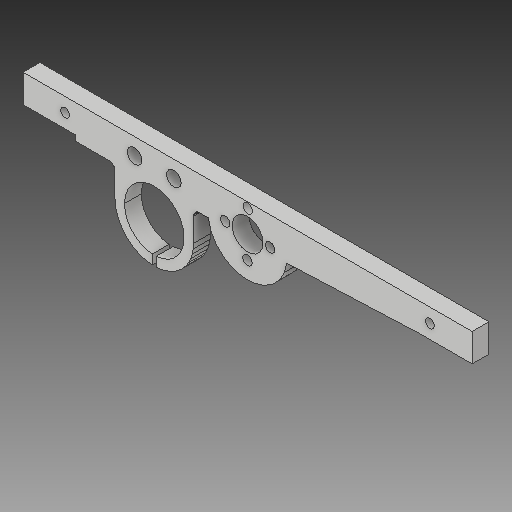
# Autodesk Inventor part: Rear-Bed-Holder-mid
Saved by Autodesk Inventor 2017 (Build 210142000, 142)
## iProperties
Created: 2016-07-12
Part Number: Rear-Bed-Holder-mid
Material: Generic
Document SubType Name: Modeling
Designer: joshmamo
Density: 1 g/cm^3
Appearance: Default
Author: joshmamo
Autodesk Inventor part; units mm, degrees
ref_plane "YZ Plane" through (0, 0, 0) normal (1, 0, 0) x (0, 1, 0)
ref_plane "XZ Plane" through (0, 0, 0) normal (0, 1, 0) x (-1, 0, 0)
ref_plane "XY Plane" through (0, 0, 0) normal (0, 0, 1) x (1, 0, 0)
sketch "Sketch1" plane through (0, 0, 0) normal (0, 0, 1) x (1, 0, 0)
  line L0 (326.8705, 297.7695) -> (327.1965, 298.0306)
  line L1 (327.1965, 298.0306) -> (327.4439, 298.3671)
  line L2 (327.4439, 298.3671) -> (327.5957, 298.7562)
  line L3 (327.5957, 298.7562) -> (327.6417, 299.1714)
  line L4 (327.6417, 299.1714) -> (327.5786, 299.5843)
  line L5 (324.4883, 299.5205) -> (324.4424, 299.1053)
  line L6 (324.4424, 299.1053) -> (324.5054, 298.6924)
  line L7 (324.5054, 298.6924) -> (324.6732, 298.3099)
  line L8 (324.6732, 298.3099) -> (324.9342, 297.9839)
  line L9 (324.9342, 297.9839) -> (325.2708, 297.7365)
  line L10 (325.2708, 297.7365) -> (325.6599, 297.5847)
  line L11 (325.6599, 297.5847) -> (326.075, 297.5387)
  line L12 (326.075, 297.5387) -> (326.4879, 297.6017)
  line L13 (326.4879, 297.6017) -> (326.8705, 297.7695)
  line L14 (327.2625, 278.7736) -> (327.5885, 279.0346)
  line L15 (327.5885, 279.0346) -> (327.8359, 279.3712)
  line L16 (327.8359, 279.3712) -> (327.9877, 279.7603)
  line L17 (327.9877, 279.7603) -> (328.0337, 280.1754)
  line L18 (328.0337, 280.1754) -> (327.9707, 280.5883)
  line L19 (327.9707, 280.5883) -> (327.8029, 280.9708)
  line L20 (327.8029, 280.9708) -> (327.5418, 281.2969)
  line L21 (327.5418, 281.2969) -> (327.2053, 281.5442)
  line L22 (327.2053, 281.5442) -> (326.8162, 281.6961)
  line L23 (326.8162, 281.6961) -> (326.401, 281.7421)
  line L24 (326.401, 281.7421) -> (325.9881, 281.679)
  line L25 (325.9881, 281.679) -> (325.6056, 281.5112)
  line L26 (325.6056, 281.5112) -> (325.2796, 281.2502)
  line L27 (325.2796, 281.2502) -> (325.0322, 280.9136)
  line L28 (325.0322, 280.9136) -> (324.8804, 280.5245)
  line L29 (324.8804, 280.5245) -> (324.8344, 280.1094)
  line L30 (324.8344, 280.1094) -> (324.8974, 279.6965)
  line L31 (324.8974, 279.6965) -> (325.0652, 279.314)
  line L32 (325.0652, 279.314) -> (325.3263, 278.9879)
  line L33 (325.3263, 278.9879) -> (325.6628, 278.7405)
  line L34 (325.6628, 278.7405) -> (326.0519, 278.5887)
  line L35 (326.0519, 278.5887) -> (326.4671, 278.5427)
  line L36 (326.4671, 278.5427) -> (326.88, 278.6058)
  line L37 (326.88, 278.6058) -> (327.2625, 278.7736)
  line L38 (262.6237, 293.8404) -> (262.7835, 294.2263)
  line L39 (262.7835, 294.2263) -> (262.838, 294.6404)
  line L40 (262.838, 294.6404) -> (262.7835, 295.0545)
  line L41 (262.7835, 295.0545) -> (262.6237, 295.4404)
  line L42 (262.6237, 295.4404) -> (262.3694, 295.7717)
  line L43 (262.3694, 295.7717) -> (262.038, 296.026)
  line L44 (262.038, 296.026) -> (261.6522, 296.1859)
  line L45 (261.6522, 296.1859) -> (261.238, 296.2404)
  line L46 (261.238, 296.2404) -> (260.8239, 296.1859)
  line L47 (260.8239, 296.1859) -> (260.438, 296.026)
  line L48 (260.438, 296.026) -> (260.1067, 295.7717)
  line L49 (260.1067, 295.7717) -> (259.8524, 295.4404)
  line L50 (259.8524, 295.4404) -> (259.6926, 295.0545)
  line L51 (259.6926, 295.0545) -> (259.638, 294.6404)
  line L52 (259.638, 294.6404) -> (259.6926, 294.2263)
  line L53 (259.6926, 294.2263) -> (259.8524, 293.8404)
  line L54 (259.8524, 293.8404) -> (260.1067, 293.509)
  line L55 (260.1067, 293.509) -> (260.438, 293.2547)
  line L56 (260.438, 293.2547) -> (260.8239, 293.0949)
  line L57 (260.8239, 293.0949) -> (261.238, 293.0404)
  line L58 (261.238, 293.0404) -> (261.6522, 293.0949)
  line L59 (261.6522, 293.0949) -> (262.038, 293.2547)
  line L60 (262.038, 293.2547) -> (262.3694, 293.509)
  line L61 (262.3694, 293.509) -> (262.6237, 293.8404)
  line L62 (390.8239, 296.1859) -> (390.438, 296.026)
  line L63 (390.438, 296.026) -> (390.1067, 295.7717)
  line L64 (390.1067, 295.7717) -> (389.8524, 295.4404)
  line L65 (389.8524, 295.4404) -> (389.6926, 295.0545)
  line L66 (389.6926, 295.0545) -> (389.638, 294.6404)
  line L67 (389.638, 294.6404) -> (389.6926, 294.2263)
  line L68 (389.6926, 294.2263) -> (389.8524, 293.8404)
  line L69 (389.8524, 293.8404) -> (390.1067, 293.509)
  line L70 (390.1067, 293.509) -> (390.438, 293.2547)
  line L71 (390.438, 293.2547) -> (390.8239, 293.0949)
  line L72 (390.8239, 293.0949) -> (391.238, 293.0404)
  line L73 (391.238, 293.0404) -> (391.6522, 293.0949)
  line L74 (391.6522, 293.0949) -> (392.038, 293.2547)
  line L75 (392.038, 293.2547) -> (392.3694, 293.509)
  line L76 (392.3694, 293.509) -> (392.6237, 293.8404)
  line L77 (392.6237, 293.8404) -> (392.7835, 294.2263)
  line L78 (392.7835, 294.2263) -> (392.838, 294.6404)
  line L79 (392.838, 294.6404) -> (392.7835, 295.0545)
  line L80 (392.7835, 295.0545) -> (392.6237, 295.4404)
  line L81 (392.6237, 295.4404) -> (392.3694, 295.7717)
  line L82 (392.3694, 295.7717) -> (392.038, 296.026)
  line L83 (392.038, 296.026) -> (391.6522, 296.1859)
  line L84 (391.6522, 296.1859) -> (391.238, 296.2404)
  line L85 (391.238, 296.2404) -> (390.8239, 296.1859)
  line L86 (318.1419, 288.6731) -> (318.2938, 289.0622)
  line L87 (318.2938, 289.0622) -> (318.3397, 289.4774)
  line L88 (318.3397, 289.4774) -> (318.2767, 289.8903)
  line L89 (318.2767, 289.8903) -> (318.1089, 290.2728)
  line L90 (318.1089, 290.2728) -> (317.8479, 290.5988)
  line L91 (317.8479, 290.5988) -> (317.5113, 290.8462)
  line L92 (317.5113, 290.8462) -> (317.1222, 290.9981)
  line L93 (317.1222, 290.9981) -> (316.7071, 291.044)
  line L94 (316.7071, 291.044) -> (316.2942, 290.981)
  line L95 (316.2942, 290.981) -> (315.9116, 290.8132)
  line L96 (315.9116, 290.8132) -> (315.5856, 290.5521)
  line L97 (315.5856, 290.5521) -> (315.3382, 290.2156)
  line L98 (315.3382, 290.2156) -> (315.1864, 289.8265)
  line L99 (315.1864, 289.8265) -> (315.1404, 289.4114)
  line L100 (315.1404, 289.4114) -> (315.2035, 288.9985)
  line L101 (315.2035, 288.9985) -> (315.3712, 288.6159)
  line L102 (315.3712, 288.6159) -> (315.6323, 288.2899)
  line L103 (315.6323, 288.2899) -> (315.9688, 288.0425)
  line L104 (315.9688, 288.0425) -> (316.3579, 287.8907)
  line L105 (316.3579, 287.8907) -> (316.7731, 287.8447)
  line L106 (316.7731, 287.8447) -> (317.186, 287.9078)
  line L107 (317.186, 287.9078) -> (317.5685, 288.0755)
  line L108 (317.5685, 288.0755) -> (317.8945, 288.3366)
  line L109 (317.8945, 288.3366) -> (318.1419, 288.6731)
  line L110 (334.1994, 289.3905) -> (334.3672, 289.008)
  line L111 (334.3672, 289.008) -> (334.6282, 288.6819)
  line L112 (334.6282, 288.6819) -> (334.9648, 288.4345)
  line L113 (334.9648, 288.4345) -> (335.3539, 288.2827)
  line L114 (335.3539, 288.2827) -> (335.769, 288.2367)
  line L115 (335.769, 288.2367) -> (336.1819, 288.2998)
  line L116 (336.1819, 288.2998) -> (336.5644, 288.4675)
  line L117 (336.5644, 288.4675) -> (336.8905, 288.7286)
  line L118 (336.8905, 288.7286) -> (337.1379, 289.0651)
  line L119 (337.1379, 289.0651) -> (337.2897, 289.4542)
  line L120 (337.2897, 289.4542) -> (337.3357, 289.8694)
  line L121 (337.3357, 289.8694) -> (337.2726, 290.2823)
  line L122 (337.2726, 290.2823) -> (337.1049, 290.6648)
  line L123 (337.1049, 290.6648) -> (336.8438, 290.9908)
  line L124 (336.8438, 290.9908) -> (336.5073, 291.2382)
  line L125 (336.5073, 291.2382) -> (336.1182, 291.3901)
  line L126 (336.1182, 291.3901) -> (335.703, 291.436)
  line L127 (335.703, 291.436) -> (335.2901, 291.373)
  line L128 (335.2901, 291.373) -> (334.9076, 291.2052)
  line L129 (334.9076, 291.2052) -> (334.5815, 290.9442)
  line L130 (334.5815, 290.9442) -> (334.3342, 290.6076)
  line L131 (334.3342, 290.6076) -> (334.1823, 290.2185)
  line L132 (334.1823, 290.2185) -> (334.1364, 289.8034)
  line L133 (334.1364, 289.8034) -> (334.1994, 289.3905)
  line L134 (324.6214, 275.5909) -> (321.0402, 276.4881)
  line L135 (321.0402, 276.4881) -> (317.8133, 278.2815)
  line L136 (317.8133, 278.2815) -> (315.1604, 280.8491)
  line L137 (315.1604, 280.8491) -> (313.2626, 284.0157)
  line L138 (313.2626, 284.0157) -> (312.2489, 287.5657)
  line L139 (312.2489, 287.5657) -> (312.2467, 287.7002)
  line L140 (312.2467, 287.7002) -> (309.0912, 287.7002)
  line L141 (309.0912, 287.7002) -> (308.7265, 287.6683)
  line L142 (308.7265, 287.6683) -> (308.373, 287.5736)
  line L143 (308.373, 287.5736) -> (308.0412, 287.4189)
  line L144 (308.0412, 287.4189) -> (307.7413, 287.2089)
  line L145 (307.7413, 287.2089) -> (307.4825, 286.9501)
  line L146 (307.4825, 286.9501) -> (307.2725, 286.6502)
  line L147 (307.2725, 286.6502) -> (307.1178, 286.3185)
  line L148 (307.1178, 286.3185) -> (307.0231, 285.9649)
  line L149 (307.0231, 285.9649) -> (306.9912, 285.6002)
  line L150 (306.9912, 285.6002) -> (306.9912, 277.2002)
  line L151 (306.9912, 277.2002) -> (306.8789, 275.4307)
  line L152 (306.8789, 275.4307) -> (306.5439, 273.6896)
  line L153 (306.5439, 273.6896) -> (305.9915, 272.0048)
  line L154 (305.9915, 272.0048) -> (305.2306, 270.4034)
  line L155 (305.2306, 270.4034) -> (304.2733, 268.9109)
  line L156 (304.2733, 268.9109) -> (303.1352, 267.5514)
  line L157 (303.1352, 267.5514) -> (301.8343, 266.3467)
  line L158 (301.8343, 266.3467) -> (300.3915, 265.316)
  line L159 (300.3915, 265.316) -> (298.8301, 264.476)
  line L160 (298.8301, 264.476) -> (297.175, 263.84)
  line L161 (297.175, 263.84) -> (295.4529, 263.4184)
  line L162 (295.4529, 263.4184) -> (293.6912, 263.2177)
  line L163 (293.6912, 263.2177) -> (293.6912, 266.7236)
  line L164 (293.6912, 266.7236) -> (295.3277, 266.9635)
  line L165 (295.3277, 266.9635) -> (296.9062, 267.4574)
  line L166 (296.9062, 267.4574) -> (298.3876, 268.1931)
  line L167 (298.3876, 268.1931) -> (299.7351, 269.1522)
  line L168 (299.7351, 269.1522) -> (300.9152, 270.3111)
  line L169 (300.9152, 270.3111) -> (301.8987, 271.6409)
  line L170 (301.8987, 271.6409) -> (302.6612, 273.1086)
  line L171 (302.6612, 273.1086) -> (303.1837, 274.6779)
  line L172 (303.1837, 274.6779) -> (303.4534, 276.3098)
  line L173 (303.4534, 276.3098) -> (303.4634, 277.9637)
  line L174 (303.4634, 277.9637) -> (303.2136, 279.5988)
  line L175 (303.2136, 279.5988) -> (302.7101, 281.1743)
  line L176 (302.7101, 281.1743) -> (301.9655, 282.6511)
  line L177 (301.9655, 282.6511) -> (300.9982, 283.9928)
  line L178 (300.9982, 283.9928) -> (299.8322, 285.1659)
  line L179 (299.8322, 285.1659) -> (298.4964, 286.1413)
  line L180 (298.4964, 286.1413) -> (297.0241, 286.8949)
  line L181 (297.0241, 286.8949) -> (295.4517, 287.4079)
  line L182 (295.4517, 287.4079) -> (293.8182, 287.6676)
  line L183 (293.8182, 287.6676) -> (292.1642, 287.6676)
  line L184 (292.1642, 287.6676) -> (290.5307, 287.4079)
  line L185 (290.5307, 287.4079) -> (288.9583, 286.8949)
  line L186 (288.9583, 286.8949) -> (287.486, 286.1413)
  line L187 (287.486, 286.1413) -> (286.1502, 285.1659)
  line L188 (286.1502, 285.1659) -> (284.9842, 283.9928)
  line L189 (284.9842, 283.9928) -> (284.0169, 282.6511)
  line L190 (284.0169, 282.6511) -> (283.2723, 281.1743)
  line L191 (283.2723, 281.1743) -> (282.7688, 279.5988)
  line L192 (282.7688, 279.5988) -> (282.519, 277.9637)
  line L193 (282.519, 277.9637) -> (282.529, 276.3098)
  line L194 (282.529, 276.3098) -> (282.7986, 274.6779)
  line L195 (282.7986, 274.6779) -> (283.3212, 273.1086)
  line L196 (283.3212, 273.1086) -> (284.0837, 271.6409)
  line L197 (284.0837, 271.6409) -> (285.0672, 270.3111)
  line L198 (285.0672, 270.3111) -> (286.2473, 269.1522)
  line L199 (286.2473, 269.1522) -> (287.5948, 268.1931)
  line L200 (287.5948, 268.1931) -> (289.0762, 267.4574)
  line L201 (289.0762, 267.4574) -> (290.6547, 266.9635)
  line L202 (290.6547, 266.9635) -> (292.2912, 266.7236)
  line L203 (292.2912, 266.7236) -> (292.2912, 263.2177)
  line L204 (292.2912, 263.2177) -> (290.5295, 263.4184)
  line L205 (290.5295, 263.4184) -> (288.8073, 263.84)
  line L206 (288.8073, 263.84) -> (287.1523, 264.476)
  line L207 (287.1523, 264.476) -> (285.5909, 265.316)
  line L208 (285.5909, 265.316) -> (284.1481, 266.3467)
  line L209 (284.1481, 266.3467) -> (282.8472, 267.5514)
  line L210 (282.8472, 267.5514) -> (281.709, 268.9109)
  line L211 (281.709, 268.9109) -> (280.7518, 270.4034)
  line L212 (280.7518, 270.4034) -> (279.9909, 272.0048)
  line L213 (279.9909, 272.0048) -> (279.4385, 273.6896)
  line L214 (279.4385, 273.6896) -> (279.1035, 275.4307)
  line L215 (279.1035, 275.4307) -> (278.9912, 277.2002)
  line L216 (278.9912, 277.2002) -> (278.9912, 285.6002)
  line L217 (278.9912, 285.6002) -> (278.9593, 285.9649)
  line L218 (278.9593, 285.9649) -> (278.8645, 286.3185)
  line L219 (278.8645, 286.3185) -> (278.7098, 286.6502)
  line L220 (278.7098, 286.6502) -> (278.4999, 286.9501)
  line L221 (278.4999, 286.9501) -> (278.241, 287.2089)
  line L222 (278.241, 287.2089) -> (277.9412, 287.4189)
  line L223 (277.9412, 287.4189) -> (277.6094, 287.5736)
  line L224 (277.6094, 287.5736) -> (277.2559, 287.6683)
  line L225 (277.2559, 287.6683) -> (276.8912, 287.7002)
  line L226 (276.8912, 287.7002) -> (264.9912, 287.7002)
  line L227 (264.9912, 287.7002) -> (264.9912, 289.6404)
  line L228 (264.9912, 289.6404) -> (246.238, 289.6404)
  line L229 (246.238, 289.6404) -> (246.238, 299.6404)
  line L230 (246.238, 299.6404) -> (406.238, 299.6404)
  line L231 (406.238, 299.6404) -> (406.238, 289.6404)
  line L232 (406.238, 289.6404) -> (387.4849, 289.6404)
  line L233 (387.4849, 289.6404) -> (340.2064, 287.7002)
  line L234 (340.2064, 287.7002) -> (339.3903, 284.4425)
  line L235 (339.3903, 284.4425) -> (337.5969, 281.2156)
  line L236 (337.5969, 281.2156) -> (335.0293, 278.5628)
  line L237 (335.0293, 278.5628) -> (331.8627, 276.6649)
  line L238 (331.8627, 276.6649) -> (328.3127, 275.6512)
  line L239 (328.3127, 275.6512) -> (324.6214, 275.5909)
  circle A0 centre (326.238, 289.6404) radius 5.5
  circle A1 centre (285.9912, 293.6676) radius 2.6
  circle A2 centre (299.9912, 293.6676) radius 2.6
  point P0 (0, 0)
  constraints: 480 end point, 3 centre point
extrude "Extrusion1" add sketch "Sketch1" along normal blind 6
sketch "Sketch2" plane through (0, 0, 6) normal (0, 0, 1) x (1, 0, 0)
  line L0 (318.3397, 289.4774) -> (318.2938, 289.0622) projected
  line L1 (315.1404, 289.4114) -> (318.3397, 289.4774)
  line L2 (334.1823, 290.2185) -> (334.1364, 289.8034) projected
  line L3 (337.2726, 290.2823) -> (337.3357, 289.8694) projected
  line L4 (334.1364, 289.8034) -> (337.3357, 289.8694)
  line L5 (318.2767, 289.8903) -> (318.3397, 289.4774) projected
  line L6 (334.1364, 289.8034) -> (318.3397, 289.4774)
  line L7 (324.8804, 280.5245) -> (324.8344, 280.1094) projected
  line L8 (328.0337, 280.1754) -> (324.8344, 280.1094)
  circle A0 centre (326.434, 280.1424) radius 1.6
  circle A1 centre (326.042, 299.1383) radius 1.6
  point P0 (0, 0)
  dimension "d2" = 3.2
  constraints: 8 end point, 2 centre point, 1 midpoint, 1 symmetric about line, 1 other
  measures "d2" diameter of A0
extrude "Extrusion2" cut sketch "Sketch2" against normal through all contours A1
sketch "Sketch3" plane through (0, 0, 6) normal (0, 0, 1) x (1, 0, 0)
  line L0 (262.7835, 295.0545) -> (262.838, 294.6404) projected
  line L1 (259.6926, 294.2263) -> (259.638, 294.6404) projected
  line L2 (262.838, 294.6404) -> (259.638, 294.6404)
  line L3 (389.638, 294.6404) -> (389.6926, 294.2263) projected
  line L4 (392.838, 294.6404) -> (389.638, 294.6404)
  point P0 (0, 0)
  point P1 (391.238, 294.6404)
  point P2 (261.238, 294.6404)
  constraints: 4 end point, 2 horizontal, 2 midpoint
hole "Hole1" at (391.238, 294.6404, 6) at (261.238, 294.6404, 6) direction (0, 0, -1) diameter 3.2 depth 8 tip angle 118
sketch "Sketch4" plane through (0, 0, 6) normal (0, 0, 1) x (1, 0, 0)
  line L0 (303.4634, 277.9637) -> (303.4534, 276.3098) projected
  line L1 (303.4584, 277.1368) -> (282.524, 277.1368)
  line L2 (282.519, 277.9637) -> (282.529, 276.3098) projected
  point P0 (0, 0)
  point P1 (292.9912, 277.1368)
  constraints: 3 midpoint, 2 end point
hole "Hole2" at (292.9912, 277.1368, 6) direction (0, 0, -1) diameter 21.2 depth 8 tip angle 118
sketch "Sketch5" plane through (0, 0, 6) normal (0, 0, 1) x (1, 0, 0)
  arc A0 (293.6912, 266.6865) -> (292.2912, 266.6865) centre (292.9912, 277.2634) ccw projected
  point P0 (0, 0)
hole "Hole3" at (292.9912, 277.2634, 6) direction (0, 0, -1) diameter 21.2 depth 8 tip angle 118
sketch "Sketch6" plane through (0, 0, 6) normal (0, 0, 1) x (1, 0, 0)
  line L0 (337.2726, 290.2823) -> (337.3357, 289.8694) projected
  line L1 (334.1994, 289.3905) -> (334.1364, 289.8034) projected
  line L2 (337.3357, 289.8694) -> (334.1364, 289.8034)
  line L3 (327.9707, 280.5883) -> (328.0337, 280.1754) projected
  line L4 (324.8344, 280.1094) -> (324.8804, 280.5245) projected
  line L5 (328.0337, 280.1754) -> (324.8344, 280.1094)
  line L6 (318.3397, 289.4774) -> (318.2938, 289.0622) projected
  line L7 (315.2035, 288.9985) -> (315.1404, 289.4114) projected
  line L8 (318.3397, 289.4774) -> (315.1404, 289.4114)
  point P0 (0, 0)
  point P1 (316.7401, 289.4444)
  point P2 (326.434, 280.1424)
  point P3 (335.736, 289.8364)
  constraints: 6 end point, 3 midpoint
hole "Hole4" at (316.7401, 289.4444, 6) at (326.434, 280.1424, 6) at (335.736, 289.8364, 6) direction (0, 0, -1) diameter 3.2 depth 8 tip angle 118
sketch "Sketch7" plane through (0, 0, 6) normal (0, 0, 1) x (1, 0, 0)
  line L0 (327.5612, 299.6404) -> (406.238, 299.6404) projected
  line L1 (327.5612, 299.6404) -> (324.4562, 299.6404)
  line L2 (324.4562, 299.6404) -> (313.5339, 291.0236)
  line L3 (313.5339, 291.0236) -> (320.8154, 278.2809)
  line L4 (320.8154, 278.2809) -> (328.6422, 276.3946)
  line L5 (328.6422, 276.3946) -> (338.6249, 286.3186)
  line L6 (338.6249, 286.3186) -> (338.2503, 292.466)
  line L7 (338.2503, 292.466) -> (333.7875, 292.466)
  line L8 (333.7875, 292.466) -> (332.6354, 287.6855)
  line L9 (332.6354, 287.6855) -> (329.7411, 283.8008)
  line L10 (329.7411, 283.8008) -> (323.1516, 282.1433)
  line L11 (323.1516, 282.1433) -> (318.6114, 290.0886)
  line L12 (318.6114, 290.0886) -> (324.7498, 296.1908)
  line L13 (324.7498, 296.1908) -> (327.8641, 297.3687)
  line L14 (327.8641, 297.3687) -> (329.6443, 299.1383)
  line L15 (329.6443, 299.1383) -> (327.5612, 299.6404)
  point P0 (0, 0)
  constraints: 30 end point, 4 parallel, 2 perpendicular, 1 horizontal
extrude "Extrusion3" add sketch "Sketch7" against normal blind 6
sketch "Sketch8" plane through (0, 0, 6) normal (0, 0, 1) x (1, 0, 0)
  circle A0 centre (326.2243, 281.6404) radius 1.7 projected
  circle A1 centre (334.2568, 289.6077) radius 1.7 projected
  circle A2 centre (326.2894, 297.6402) radius 1.7 projected
  circle A3 centre (318.2569, 289.6728) radius 1.7 projected
  point P0 (0, 0)
extrude "Extrusion4" cut sketch "Sketch8" against normal blind 6
body "Solid1"
